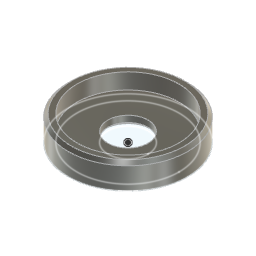
_32mm Magnet Base.29063411-a0db-4089-ad1e-33dbe9d709d5 (Autodesk Fusion 360 design; units mm, degrees)
Autodesk Fusion 360 part; units mm, degrees
sketch "Sketch1" plane through (0, 0, 0) normal (0, 0, 1) x (1, 0, 0)
  circle A0 centre (0, 0) radius 16.25
  circle A1 centre (0, 0) radius 19
  circle A2 centre (0, 0) radius 6.4
  dimension "d1" = 32.5
  dimension "d2" = 38
  dimension "d3" = 12.8
  constraint coincident A0.centre A1.centre
  constraint concentric A0 A1
  constraint concentric A0 A2
  measures "d1" diameter of A0
  measures "d2" diameter of A1
  measures "d3" diameter of A2
extrude "Extrude1" add sketch "Sketch1" along normal blind 8 contours A1
extrude "Extrude2" add sketch "Sketch1" along normal blind 3 contours A0
chamfer "Chamfer1" distance 1 angle 45 1 edges at (-17.7142, -6.8707, 8)
chamfer "Chamfer2" distance 1 angle 45 1 edges at (-5.9669, 2.3143, 0)
